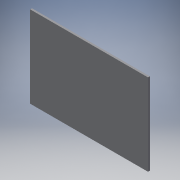
# Autodesk Inventor part: Платформа
Saved by Autodesk Inventor 2018 (Build 220112000, 112)
## iProperties
Created: 2023-02-19
Part Number: Платформа
Material: Типовые
Document SubType Name: Modeling
Designer: exper
Density: 1 g/cm^3
Appearance: По умолчанию
Author: exper
Autodesk Inventor part; units mm, degrees
ref_plane "YZ Plane" through (0, 0, 0) normal (1, 0, 0) x (0, 1, 0)
ref_plane "XZ Plane" through (0, 0, 0) normal (0, 1, 0) x (-1, 0, 0)
ref_plane "XY Plane" through (0, 0, 0) normal (0, 0, 1) x (1, 0, 0)
sketch "Эскиз1" plane through (0, 0, 0) normal (0, 1, 0) x (-1, 0, 0)
  line L0 (0, 0) -> (-375, 0)
  line L1 (-375, 0) -> (-375, -260)
  line L2 (-375, -260) -> (0, -260)
  line L3 (0, -260) -> (0, 0)
  dimension "d0" = 375
  dimension "d1" = 260
  constraints: 8 end point, 2 parallel, 1 horizontal, 1 perpendicular
  measures "d0" distance of L2.end L1.end
  measures "d1" distance of L1.end L0.end
extrude "Выдавливание1" add sketch "Эскиз1" along normal blind 6
